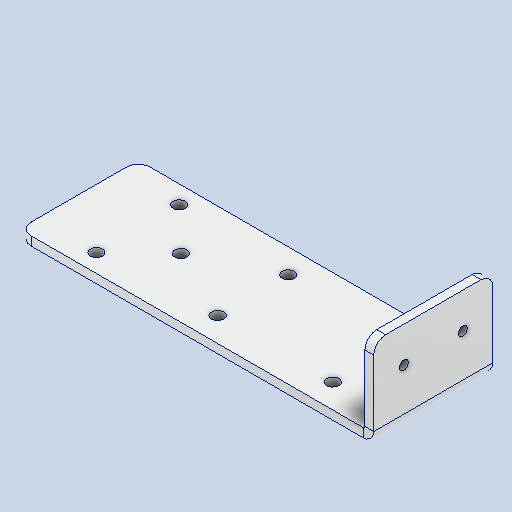
# Autodesk Inventor part: servo-horn_top
Saved by Autodesk Inventor 2023 (Build 270158000, 158)
## iProperties
Created: 2022-10-09
Part Number: servo-horn_top
Material: 알루미늄 6061
Document SubType Name: Sheet Metal
Designer: 박동준
Density: 2.7 g/cm^3
Sheet Metal Rule: Default_mm
Appearance: 알루미늄 - 평지
Flat Pattern Width: 2.014 cm
Flat Pattern Length: 7.22793 cm
Flat Pattern Area: 14.557 cm^2
Sheet Metal Width: 20.140 mm
Sheet Metal Length: 72.279 mm
Sheet Metal Area: 1455.705 mm^2
품번: 17
Author: 박동준
Autodesk Inventor part; units mm, degrees
ref_plane "YZ Plane" through (0, 0, 0) normal (1, 0, 0) x (0, 1, 0)
ref_plane "XZ Plane" through (0, 0, 0) normal (0, 1, 0) x (-1, 0, 0)
ref_plane "XY Plane" through (0, 0, 0) normal (0, 0, 1) x (1, 0, 0)
sketch "스케치1" plane through (0, 0, 0) normal (0, 1, 0) x (-1, 0, 0)
  line L0 (30, -10.07) -> (-30, -10.07)
  line L1 (-30, -10.07) -> (-30, 10.07)
  line L2 (-30, 10.07) -> (30, 10.07)
  line L3 (30, 10.07) -> (30, -10.07)
  point P0 (0, 0)
  point P1 (0, -10.07)
  point P2 (30, 0)
  dimension "d0" = 20.14
  dimension "d1" = 60
  measures "d0" distance between parallel lines of L2 L0
  measures "d1" distance of L0.start L0.end
extrude "판1" add sketch "스케치1" along normal mid plane 1.5
sketch "스케치2" plane through (28.5, -0.75, -10.07) normal (1, 0, 0) x (0, 1, 0)
  line L0 (0, 20.14) -> (0, 0)
  line L1 (0, 0) -> (15, 0)
  line L2 (15, 0) -> (15, 20.14)
  line L3 (15, 20.14) -> (0, 20.14)
  constraints: 6 end point, 1 horizontal, 1 perpendicular, 1 vertical
edge flange "플랜지1" height 15 angle 90 thickness 1.5 bend radius 0.31 thickness toward (1, 0, 0) relief tear relief width 1.5 relief depth 0.75 edges at (30, 0.75, 0) wall of the first edge with corners at (28.5, -0.75, 10.07) (28.5, -0.75, -10.07) (28.5, 14.25, -10.07) (28.5, 14.25, 10.07)
bend "절곡부1"
corner "구석1"
sketch "스케치3" plane through (0, 0.75, 0) normal (0, 1, 0) x (1, 0, 0)
  line L0 (-30, -10.07) -> (-30, 10.07) projected
  line L1 (-20, 7) -> (-20, -7) construction
  circle A0 centre (-20, 7) radius 1.05
  circle A1 centre (-12.7, 0) radius 1.05
  circle A2 centre (-20, -7) radius 1.05
  point P0 (0, 0)
  point P1 (-20, 0)
  dimension "d14" = 10
  dimension "d15" = 10
  dimension "d16" = 14
  dimension "d17" = 7.3
  dimension "d18" = 2.1
  dimension "d19" = 2.1
  dimension "d20" = 2.1
  constraints: 3 centre point, 3 coincident, 2 end point, 2 horizontal alignment, 1 midpoint
  measures "d14" distance from line of L0 L1.start
  measures "d15" distance from line of L0 L1.end
  measures "d16" distance of L1.end L1.start
  measures "d17" horizontal distance of point (-12.7, 0) L1.start
  measures "d18" diameter of A0
  measures "d19" diameter of A1
  measures "d20" diameter of A2
extrude "돌출1" cut sketch "스케치3" against normal through all
sketch "스케치4" plane through (30, 14.25, 10.07) normal (1, 0, 0) x (0, 0, -1)
  line L0 (0, 0) -> (20.14, 0) projected
  line L1 (5.07, -6) -> (15.07, -6) construction
  point P0 (10.07, -14.25)
  point P1 (10.07, 0)
  point P2 (10.07, 0)
  point P3 (10.07, 0)
  point P4 (10.07, -6)
  point P5 (10.07, 0)
  point P6 (10.07, 0)
  dimension "d34" = 10
  dimension "d35" = 6
  constraints: 6 midpoint, 2 coincident, 2 end point, 1 horizontal, 1 vertical alignment
  measures "d34" distance of L1.start L1.end
  measures "d35" distance of point (10.07, -6) point (10.07, 0)
fillet "모깎기1" radius 2 4 edges at (29.25, 14.25, 10.07) (29.25, 14.25, -10.07) (-30, 0, 10.07) (-30, 0, -10.07)
hole "구멍1" at (30, 8.25, 5) at (30, 8.25, -5) direction (-1, 0, 0) diameter 1.567 end through all thread size "M2x0.4" class "6H" standard "ISO Metric profile"
sketch "Sketch5" plane through (0, -0.75, 0) normal (0, -1, 0) x (1, 0, 0)
  circle A0 centre (-0.52, 5.975) radius 0.7835 projected
  circle A1 centre (18.98, 5.975) radius 0.7835 projected
  circle A2 centre (-0.52, 5.975) radius 1.05
  circle A3 centre (18.98, 5.975) radius 1.05
  circle A4 centre (-12.7, 0) radius 1.05 projected
  circle A5 centre (-20, -7) radius 1.05 projected
  circle A6 centre (-20, 7) radius 1.05 projected
  arc A7 (-30, -8.07) -> (-28, -10.07) centre (-28, -8.07) ccw projected
  line L0 (-28, -10.07) -> (28.19, -10.07) projected
  line L1 (28.19, -10.07) -> (28.19, 10.07) projected
  line L2 (28.19, 10.07) -> (-28, 10.07) projected
  arc A8 (-28, 10.07) -> (-30, 8.07) centre (-28, 8.07) ccw projected
  line L3 (-30, 8.07) -> (-30, -8.07) projected
  line L4 (-30, 0) -> (28.19, 0) construction
  circle A9 centre (-0.52, -5.975) radius 1.05
  circle A10 centre (18.98, -5.975) radius 1.05
  point P0 (0, 0)
  dimension "d43" = 2.1
  constraints: 4 centre point, 2 coincident, 2 end point, 2 midpoint, 2 symmetric about line, 1 equal radius, 2 other
  measures "d43" diameter of A2
extrude "Cut1" cut sketch "Sketch5" against normal blind 1.5 contours A0 | A1 | A2 | A3 | A9 | A10
equation "\"d3\" = BendReliefWidth"
equation "\"d4\" = BendReliefDepth"
equation "\"d5\" = MinimumRemnant"
equation "\"d6\" = TransitionRadius"
equation "\"d10\" = CornerReliefSize"
equation "\"TransitionRadius\" = BendRadius"
equation "\"BendReliefWidth\" = 1.5"
equation "\"BendReliefDepth\" = 0.75"
equation "\"MinimumRemnant\" = 3"
equation "\"CornerReliefSize\" = 6"
equation "\"BendRadius\" = 0.31"
